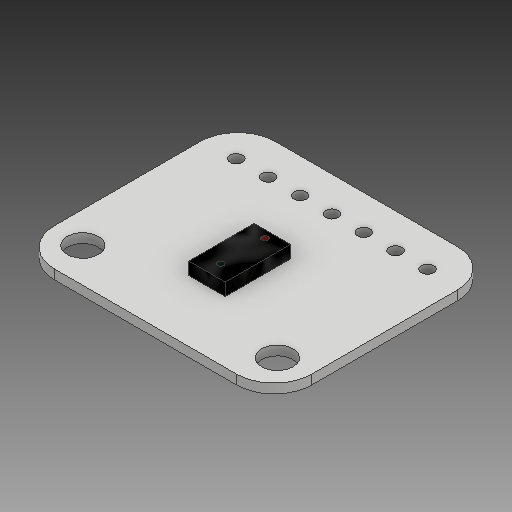
# Autodesk Inventor part: VL6180X-Time_of_Flight_Sensor
Saved by Autodesk Inventor 2018 (Build 220112000, 112)
## iProperties
Part Number: VL6180X-Time_of_Flight_Sensor
Material: Generisch
Document SubType Name: Modeling
Designer: Jochen Alt
Mass: 0.268007 g
Surface Area: 7.76421 cm^2
Volume: 0.268007 cm^3
Density: 1 g/cm^3
Appearance: Vorgabe
Author: Jochen Alt
Autodesk Inventor part; units mm, degrees
ref_plane "YZ Plane" through (0, 0, 0) normal (1, 0, 0) x (0, 1, 0)
ref_plane "XZ Plane" through (0, 0, 0) normal (0, 1, 0) x (-1, 0, 0)
ref_plane "XY Plane" through (0, 0, 0) normal (0, 0, 1) x (1, 0, 0)
sketch "Skizze1" plane through (0, 0, 0) normal (0, 0, 1) x (1, 0, 0)
  line L0 (-10.25, -8.8) -> (10.25, -8.8)
  line L1 (10.25, -8.8) -> (10.25, 8.8)
  line L2 (10.25, 8.8) -> (-10.25, 8.8)
  line L3 (-10.25, 8.8) -> (-10.25, -8.8)
  line L4 (-10.25, -8.8) -> (10.25, 8.8) construction
  line L5 (10.25, -8.8) -> (-10.25, 8.8) construction
  point P0 (0, 0)
  dimension "d0" = 20.5
  dimension "d1" = 17.6
  constraints: 12 end point, 2 midpoint, 2 parallel, 1 horizontal, 1 perpendicular
  measures "d0" distance of L2.end L1.end
  measures "d1" distance of L1.end L0.end
extrude "Extrusion1" add sketch "Skizze1" along normal blind 0.75
fillet "Rundung1" radius 3 4 edges at (10.25, -8.8, 0.375) (-10.25, -8.8, 0.375) (-10.25, 8.8, 0.375) (10.25, 8.8, 0.375)
sketch "Skizze2" plane through (0, 0, 0.75) normal (0, 0, 1) x (1, 0, 0)
  line L0 (7.75, -6.05) -> (-7.75, -6.05) construction
  line L1 (-7.75, -6.05) -> (-7.75, 6.05) construction
  line L2 (-7.75, 6.05) -> (7.75, 6.05) construction
  line L3 (7.75, 6.05) -> (7.75, -6.05) construction
  line L4 (7.75, -6.05) -> (-7.75, 6.05) construction
  line L5 (-7.75, -6.05) -> (7.75, 6.05) construction
  circle A0 centre (-7.75, -6.05) radius 1.25
  circle A1 centre (7.75, -6.05) radius 1.25
  line L6 (-15.2198, 0) -> (15.2198, 0) construction
  circle A2 centre (0, 6.05) radius 0.5
  line L7 (-5.21, 6.05) -> (10.29, 6.05) construction
  circle A3 centre (2.54, 6.05) radius 0.5
  line L8 (-2.67, 6.05) -> (12.83, 6.05) construction
  circle A4 centre (5.08, 6.05) radius 0.5
  line L9 (-0.13, 6.05) -> (15.37, 6.05) construction
  circle A5 centre (7.62, 6.05) radius 0.5
  line L10 (-10.29, 6.05) -> (5.21, 6.05) construction
  circle A6 centre (-2.54, 6.05) radius 0.5
  line L11 (-7.75, 6.05) -> (7.75, 6.05) construction
  circle A7 centre (0, 6.05) radius 0.5
  line L12 (-5.21, 6.05) -> (10.29, 6.05) construction
  circle A8 centre (2.54, 6.05) radius 0.5
  line L13 (-2.67, 6.05) -> (12.83, 6.05) construction
  circle A9 centre (5.08, 6.05) radius 0.5
  line L14 (-12.83, 6.05) -> (2.67, 6.05) construction
  circle A10 centre (-5.08, 6.05) radius 0.5
  line L15 (-10.29, 6.05) -> (5.21, 6.05) construction
  circle A11 centre (-2.54, 6.05) radius 0.5
  line L16 (-7.75, 6.05) -> (7.75, 6.05) construction
  circle A12 centre (0, 6.05) radius 0.5
  line L17 (-5.21, 6.05) -> (10.29, 6.05) construction
  circle A13 centre (2.54, 6.05) radius 0.5
  line L18 (-15.37, 6.05) -> (0.13, 6.05) construction
  circle A14 centre (-7.62, 6.05) radius 0.5
  line L19 (-12.83, 6.05) -> (2.67, 6.05) construction
  circle A15 centre (-5.08, 6.05) radius 0.5
  line L20 (-10.29, 6.05) -> (5.21, 6.05) construction
  circle A16 centre (-2.54, 6.05) radius 0.5
  line L21 (-7.75, 6.05) -> (7.75, 6.05) construction
  circle A17 centre (0, 6.05) radius 0.5
  point P0 (0, 0)
  dimension "d5" = 15.5
  dimension "d6" = 12.1
  dimension "d7" = 2.5
  dimension "d10" = 1
  dimension "d13" = 2.54
  dimension "d16" = 2.54
  constraints: 42 end point, 18 centre point, 3 horizontal, 3 midpoint, 2 collinear, 2 parallel, 1 coincident, 1 equal radius, 1 perpendicular, 73 other
  measures "d5" distance of L1.end L2.end
  measures "d6" distance of L0.end L1.end
  measures "d7" diameter of A0
  measures "d10" diameter of A2
  measures "d13" distance of A2.centre A3.centre
  measures "d16" distance of A2.centre A6.centre
extrude "Extrusion2" cut sketch "Skizze2" against normal through all
sketch "Skizze3" plane through (0, 0, 0.75) normal (0, 0, 1) x (1, 0, 0)
  line L0 (-1.45, -3.9) -> (1.45, -3.9)
  line L1 (1.45, -3.9) -> (1.45, 1.3)
  line L2 (1.45, 1.3) -> (-1.45, 1.3)
  line L3 (-1.45, 1.3) -> (-1.45, -3.9)
  line L4 (-1.45, -3.9) -> (1.45, 1.3) construction
  line L5 (1.45, -3.9) -> (-1.45, 1.3) construction
  line L6 (0, -13.1898) -> (0, 13.1898) construction
  circle A0 centre (0, -2.8) radius 0.25
  circle A1 centre (0, 0.7) radius 0.25
  line L7 (-15.2198, 0) -> (15.2198, 0) construction
  point P0 (0, 0)
  point P1 (0, -1.3)
  point P2 (0, -1.3)
  dimension "d21" = 2.9
  dimension "d22" = 5.2
  dimension "d23" = 0.5
  dimension "d24" = 0.5
  dimension "d25" = 0.6
  dimension "d26" = 1.1
  dimension "d27" = 1.3
  constraints: 12 end point, 3 midpoint, 3 point on line, 2 centre point, 2 parallel, 1 horizontal, 1 perpendicular
  measures "d21" distance of L2.end L1.end
  measures "d22" distance of L1.end L0.end
  measures "d23" diameter of A0
  measures "d24" diameter of A1
  measures "d25" distance from line of A1.centre L2
  measures "d26" distance from line of L0 A0.centre
  measures "d27" distance between parallel lines of L7 L2
extrude "Extrusion3" add sketch "Skizze3" along normal blind 1
